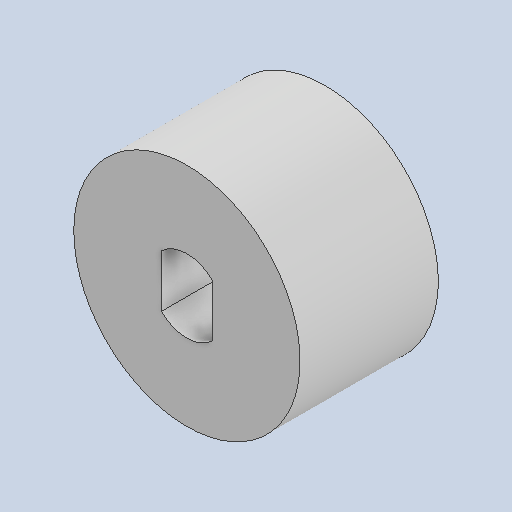
# Autodesk Inventor part: kokoko
Saved by Autodesk Inventor 2022.3 (Build 263350000, 350)
## iProperties
Created: 2023-01-17
Part Number: kokoko
Material: Generic
Document SubType Name: Modeling
Designer: komputer
Density: 1 g/cm^3
Appearance: Default
Author: komputer
Autodesk Inventor part; units mm, degrees
ref_plane "YZ Plane" through (0, 0, 0) normal (1, 0, 0) x (0, 1, 0)
ref_plane "XZ Plane" through (0, 0, 0) normal (0, 1, 0) x (-1, 0, 0)
ref_plane "XY Plane" through (0, 0, 0) normal (0, 0, 1) x (1, 0, 0)
sketch "Sketch1" plane through (0, 0, 0) normal (0, 0, 1) x (1, 0, 0)
  line L0 (0.2752, -3.536) -> (0.7321, -4.3005) projected
  arc A0 (0.5159, -4.5981) -> (0.7321, -4.3005) centre (0.5604, -4.4031) ccw projected
  line L1 (0.5159, -4.5981) -> (-0.3524, -4.3999) projected
  arc A1 (-0.3524, -4.3999) -> (-0.5862, -4.6595) centre (-0.3969, -4.5949) ccw projected
  line L2 (-0.5862, -4.6595) -> (-0.2983, -5.5023) projected
  arc A2 (-0.5716, -5.7484) -> (-0.2983, -5.5023) centre (-0.4875, -5.5669) ccw projected
  line L3 (-0.5716, -5.7484) -> (-1.3796, -5.374) projected
  arc A3 (-1.3796, -5.374) -> (-1.6623, -5.5793) centre (-1.4637, -5.5554) ccw projected
  line L4 (-1.6623, -5.5793) -> (-1.5559, -6.4635) projected
  arc A4 (-1.8745, -6.6475) -> (-1.5559, -6.4635) centre (-1.7545, -6.4874) ccw projected
  line L5 (-1.8745, -6.6475) -> (-2.587, -6.1132) projected
  arc A5 (-2.587, -6.1132) -> (-2.9062, -6.2553) centre (-2.707, -6.2732) ccw projected
  line L6 (-2.9062, -6.2553) -> (-2.9859, -7.1423) projected
  arc A6 (-3.3358, -7.256) -> (-2.9859, -7.1423) centre (-3.1851, -7.1244) ccw projected
  line L7 (-3.3358, -7.256) -> (-3.9217, -6.5853) projected
  arc A7 (-3.9217, -6.5853) -> (-4.2634, -6.6579) centre (-4.0723, -6.7169) ccw projected
  line L8 (-4.2634, -6.6579) -> (-4.5259, -7.5089) projected
  arc A8 (-4.8917, -7.5474) -> (-4.5259, -7.5089) centre (-4.717, -7.45) ccw projected
  line L9 (-4.8917, -7.5474) -> (-5.3253, -6.7695) projected
  arc A9 (-5.3253, -6.7695) -> (-5.6747, -6.7695) centre (-5.5, -6.8669) ccw projected
  line L10 (-5.6747, -6.7695) -> (-6.1083, -7.5474) projected
  arc A10 (-6.4741, -7.5089) -> (-6.1083, -7.5474) centre (-6.283, -7.45) ccw projected
  line L11 (-6.4741, -7.5089) -> (-6.7366, -6.6579) projected
  arc A11 (-6.7366, -6.6579) -> (-7.0783, -6.5853) centre (-6.9277, -6.7169) ccw projected
  line L12 (-7.0783, -6.5853) -> (-7.6642, -7.256) projected
  arc A12 (-8.0141, -7.1423) -> (-7.6642, -7.256) centre (-7.8149, -7.1244) ccw projected
  line L13 (-8.0141, -7.1423) -> (-8.0938, -6.2553) projected
  arc A13 (-8.0938, -6.2553) -> (-8.413, -6.1132) centre (-8.293, -6.2732) ccw projected
  line L14 (-8.413, -6.1132) -> (-9.1255, -6.6475) projected
  arc A14 (-9.4441, -6.4635) -> (-9.1255, -6.6475) centre (-9.2455, -6.4874) ccw projected
  line L15 (-9.4441, -6.4635) -> (-9.3377, -5.5793) projected
  arc A15 (-9.3377, -5.5793) -> (-9.6204, -5.374) centre (-9.5363, -5.5554) ccw projected
  line L16 (-9.6204, -5.374) -> (-10.4284, -5.7484) projected
  arc A16 (-10.7017, -5.5023) -> (-10.4284, -5.7484) centre (-10.5125, -5.5669) ccw projected
  line L17 (-10.7017, -5.5023) -> (-10.4138, -4.6595) projected
  arc A17 (-10.4138, -4.6595) -> (-10.6476, -4.3999) centre (-10.6031, -4.5949) ccw projected
  line L18 (-10.6476, -4.3999) -> (-11.5159, -4.5981) projected
  arc A18 (-11.7321, -4.3005) -> (-11.5159, -4.5981) centre (-11.5604, -4.4031) ccw projected
  line L19 (-11.7321, -4.3005) -> (-11.2752, -3.536) projected
  arc A19 (-11.2752, -3.536) -> (-11.4499, -3.2335) centre (-11.4469, -3.4335) ccw projected
  line L20 (-11.4499, -3.2335) -> (-12.3404, -3.2469) projected
  arc A20 (-12.49, -2.9108) -> (-12.3404, -3.2469) centre (-12.3434, -3.0469) ccw projected
  line L21 (-12.49, -2.9108) -> (-11.8842, -2.258) projected
  arc A21 (-11.8842, -2.258) -> (-11.9922, -1.9258) centre (-12.0308, -2.122) ccw projected
  line L22 (-11.9922, -1.9258) -> (-12.866, -1.7537) projected
  arc A22 (-12.9425, -1.3939) -> (-12.866, -1.7537) centre (-12.8273, -1.5575) ccw projected
  line L23 (-12.9425, -1.3939) -> (-12.2142, -0.8813) projected
  arc A23 (-12.2142, -0.8813) -> (-12.2507, -0.5339) centre (-12.3293, -0.7178) ccw projected
  line L24 (-12.2507, -0.5339) -> (-13.0696, -0.1839) projected
  arc A24 (-13.0696, 0.1839) -> (-13.0696, -0.1839) centre (-12.991, 0) ccw projected
  line L25 (-13.0696, 0.1839) -> (-12.2507, 0.5339) projected
  arc A25 (-12.2507, 0.5339) -> (-12.2142, 0.8813) centre (-12.3293, 0.7178) ccw projected
  line L26 (-12.2142, 0.8813) -> (-12.9425, 1.3939) projected
  arc A26 (-12.866, 1.7537) -> (-12.9425, 1.3939) centre (-12.8273, 1.5575) ccw projected
  line L27 (-12.866, 1.7537) -> (-11.9922, 1.9258) projected
  arc A27 (-11.9922, 1.9258) -> (-11.8842, 2.258) centre (-12.0308, 2.122) ccw projected
  line L28 (-11.8842, 2.258) -> (-12.49, 2.9108) projected
  arc A28 (-12.3404, 3.2469) -> (-12.49, 2.9108) centre (-12.3434, 3.0469) ccw projected
  line L29 (-12.3404, 3.2469) -> (-11.4499, 3.2335) projected
  arc A29 (-11.4499, 3.2335) -> (-11.2752, 3.536) centre (-11.4469, 3.4335) ccw projected
  line L30 (-11.2752, 3.536) -> (-11.7321, 4.3005) projected
  arc A30 (-11.5159, 4.5981) -> (-11.7321, 4.3005) centre (-11.5604, 4.4031) ccw projected
  line L31 (-11.5159, 4.5981) -> (-10.6476, 4.3999) projected
  arc A31 (-10.6476, 4.3999) -> (-10.4138, 4.6595) centre (-10.6031, 4.5949) ccw projected
  line L32 (-10.4138, 4.6595) -> (-10.7017, 5.5023) projected
  arc A32 (-10.4284, 5.7484) -> (-10.7017, 5.5023) centre (-10.5125, 5.5669) ccw projected
  line L33 (-10.4284, 5.7484) -> (-9.6204, 5.374) projected
  arc A33 (-9.6204, 5.374) -> (-9.3377, 5.5793) centre (-9.5363, 5.5554) ccw projected
  line L34 (-9.3377, 5.5793) -> (-9.4441, 6.4635) projected
  arc A34 (-9.1255, 6.6475) -> (-9.4441, 6.4635) centre (-9.2455, 6.4874) ccw projected
  line L35 (-9.1255, 6.6475) -> (-8.413, 6.1132) projected
  arc A35 (-8.413, 6.1132) -> (-8.0938, 6.2553) centre (-8.293, 6.2732) ccw projected
  line L36 (-8.0938, 6.2553) -> (-8.0141, 7.1423) projected
  arc A36 (-7.6642, 7.256) -> (-8.0141, 7.1423) centre (-7.8149, 7.1244) ccw projected
  line L37 (-7.6642, 7.256) -> (-7.0783, 6.5853) projected
  arc A37 (-7.0783, 6.5853) -> (-6.7366, 6.6579) centre (-6.9277, 6.7169) ccw projected
  line L38 (-6.7366, 6.6579) -> (-6.4741, 7.5089) projected
  arc A38 (-6.1083, 7.5474) -> (-6.4741, 7.5089) centre (-6.283, 7.45) ccw projected
  line L39 (-6.1083, 7.5474) -> (-5.6747, 6.7695) projected
  arc A39 (-5.6747, 6.7695) -> (-5.3253, 6.7695) centre (-5.5, 6.8669) ccw projected
  line L40 (-5.3253, 6.7695) -> (-4.8917, 7.5474) projected
  arc A40 (-4.5259, 7.5089) -> (-4.8917, 7.5474) centre (-4.717, 7.45) ccw projected
  line L41 (-4.5259, 7.5089) -> (-4.2634, 6.6579) projected
  arc A41 (-4.2634, 6.6579) -> (-3.9217, 6.5853) centre (-4.0723, 6.7169) ccw projected
  line L42 (-3.9217, 6.5853) -> (-3.3358, 7.256) projected
  arc A42 (-2.9859, 7.1423) -> (-3.3358, 7.256) centre (-3.1851, 7.1244) ccw projected
  line L43 (-2.9859, 7.1423) -> (-2.9062, 6.2553) projected
  arc A43 (-2.9062, 6.2553) -> (-2.587, 6.1132) centre (-2.707, 6.2732) ccw projected
  line L44 (-2.587, 6.1132) -> (-1.8745, 6.6475) projected
  arc A44 (-1.5559, 6.4635) -> (-1.8745, 6.6475) centre (-1.7545, 6.4874) ccw projected
  line L45 (-1.5559, 6.4635) -> (-1.6623, 5.5793) projected
  arc A45 (-1.6623, 5.5793) -> (-1.3796, 5.374) centre (-1.4637, 5.5554) ccw projected
  line L46 (-1.3796, 5.374) -> (-0.5716, 5.7484) projected
  arc A46 (-0.2983, 5.5023) -> (-0.5716, 5.7484) centre (-0.4875, 5.5669) ccw projected
  line L47 (-0.2983, 5.5023) -> (-0.5862, 4.6595) projected
  arc A47 (-0.5862, 4.6595) -> (-0.3524, 4.3999) centre (-0.3969, 4.5949) ccw projected
  line L48 (-0.3524, 4.3999) -> (0.5159, 4.5981) projected
  arc A48 (0.7321, 4.3005) -> (0.5159, 4.5981) centre (0.5604, 4.4031) ccw projected
  line L49 (0.7321, 4.3005) -> (0.2752, 3.536) projected
  arc A49 (0.2752, 3.536) -> (0.4499, 3.2335) centre (0.4469, 3.4335) ccw projected
  line L50 (0.4499, 3.2335) -> (1.3404, 3.2469) projected
  arc A50 (1.49, 2.9108) -> (1.3404, 3.2469) centre (1.3434, 3.0469) ccw projected
  line L51 (1.49, 2.9108) -> (0.8842, 2.258) projected
  arc A51 (0.8842, 2.258) -> (0.9922, 1.9258) centre (1.0308, 2.122) ccw projected
  line L52 (0.9922, 1.9258) -> (1.866, 1.7537) projected
  arc A52 (1.9425, 1.3939) -> (1.866, 1.7537) centre (1.8273, 1.5575) ccw projected
  line L53 (1.9425, 1.3939) -> (1.2142, 0.8813) projected
  arc A53 (1.2142, 0.8813) -> (1.2507, 0.5339) centre (1.3293, 0.7178) ccw projected
  line L54 (1.2507, 0.5339) -> (2.0696, 0.1839) projected
  arc A54 (2.0696, -0.1839) -> (2.0696, 0.1839) centre (1.991, 0) ccw projected
  line L55 (2.0696, -0.1839) -> (1.2507, -0.5339) projected
  arc A55 (1.2507, -0.5339) -> (1.2142, -0.8813) centre (1.3293, -0.7178) ccw projected
  line L56 (1.2142, -0.8813) -> (1.9425, -1.3939) projected
  arc A56 (1.866, -1.7537) -> (1.9425, -1.3939) centre (1.8273, -1.5575) ccw projected
  line L57 (1.866, -1.7537) -> (0.9922, -1.9258) projected
  arc A57 (0.9922, -1.9258) -> (0.8842, -2.258) centre (1.0308, -2.122) ccw projected
  line L58 (0.8842, -2.258) -> (1.49, -2.9108) projected
  arc A58 (1.3404, -3.2469) -> (1.49, -2.9108) centre (1.3434, -3.0469) ccw projected
  line L59 (1.3404, -3.2469) -> (0.4499, -3.2335) projected
  arc A59 (0.4499, -3.2335) -> (0.2752, -3.536) centre (0.4469, -3.4335) ccw projected
  circle A60 centre (-5.5, 0) radius 5.5 projected
  circle A61 centre (-5.5, 0) radius 5.5 projected
  circle A62 centre (-5.5, 0) radius 3.15 projected
  line L60 (-5.5, 0) -> (-4.6961, -7.6489)
  line L61 (-4.6961, -7.6489) -> (-4.5915, -8.6434)
  circle A63 centre (-5.5, 0) radius 8.691
  line L62 (-7.35, -1.8974) -> (-7.35, 1.8974) projected
  arc A64 (-7.35, -1.8974) -> (-3.65, -1.8974) centre (-5.5, 0) ccw projected
  line L63 (-3.65, 1.8974) -> (-3.65, -1.8974) projected
  arc A65 (-3.65, 1.8974) -> (-7.35, 1.8974) centre (-5.5, 0) ccw projected
  circle A66 centre (-5.5, 0) radius 1 projected
  point P0 (0, 0)
  dimension "d0" = 1
  constraints: 4 end point, 2 horizontal alignment, 1 coincident, 1 point on circle, 1 point on line, 3 other
  measures "d0" distance of L60.end L61.end
extrude "Extrusion1" add sketch "Sketch1" along normal blind 10 contours A63 | A62 | A60 | L0 A0 L1 A1 L2 A2 L3 A3 L4 A4 L5 A5 L6 A6 L7 A7 L8 A8 L9 A9 L10 A10 L11 A11 L12 A12 L13 A13 L14 A14 L15 A15 L16 A16 L17 A17 L18 A18 L19 A19 L20 A20 L21 A21 L22 A22 L23 A23 L24 A24 L25 A25 L26 A26 L27 A27 L28 A28 L29 A29 L30 A30 L31 A31 L32 A32 L33 A33 L34 A34 L35 A35 L36 A36 L37 A37 L38 A38 L39 A39 L40 A40 L41 A41 L42 A42 L43 A43 L44 A44 L45 A45 L46 A46 L47 A47 L48 A48 L49 A49 L50 A50 L51 A51 L52 A52 L53 A53 L54 A54 L55 A55 L56 A56 L57 A57 L58 A58 L59 A59
sketch "Sketch2" plane through (-5.5, 0, 0) normal (0, 0, -1) x (-1, 0, 0)
  circle A0 centre (0, 0) radius 8.691 projected
  arc A1 (-1.85, -1.8974) -> (1.85, -1.8974) centre (0, 0) ccw projected
  line L0 (-1.85, 1.8974) -> (-1.85, -1.8974) projected
  arc A2 (1.85, 1.8974) -> (-1.85, 1.8974) centre (0, 0) ccw projected
  line L1 (1.85, -1.8974) -> (1.85, 1.8974) projected
  circle A3 centre (0, 0) radius 8.691 projected
  line L2 (0, -8.691) -> (0, -8.191)
  circle A4 centre (0, 0) radius 8.191
  point P0 (-5.5, 0)
  dimension "d3" = 0.5
  constraints: 2 end point, 2 vertical alignment, 1 coincident, 1 vertical, 3 other
  measures "d3" distance of L2.start L2.end
extrude "Extrusion2" cut sketch "Sketch2" against normal through all contours A0
body "Solid1"
